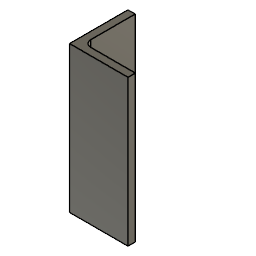
L-40×40×5 (Autodesk Fusion 360 design; units mm, degrees)
Autodesk Fusion 360 part; units mm, degrees
sketch "スケッチ1" plane through (0, 0, 0) normal (0, 0, 1) x (1, 0, 0)
  line L0 (0, 40) -> (0, 0)
  line L1 (5, 9.5) -> (5, 40)
  line L2 (40, 5) -> (9.5, 5)
  line L3 (0, 0) -> (40, 0)
  arc A0 (5, 9.5) -> (9.5, 5) centre (9.5, 9.5) ccw
  line L4 (40, 0) -> (40, 5)
  line L5 (5, 40) -> (0, 40)
extrude "押し出し1" add sketch "スケッチ1" along normal blind 100
